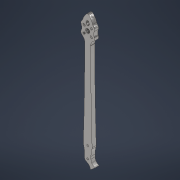
# Autodesk Inventor part: 10inchreararm
Saved by Autodesk Inventor 2021 (Build 250183000, 183)
## iProperties
Created: 2020-05-02
Part Number: 10inchreararm
Material: Generic
Document SubType Name: Modeling
Designer: Logan
Density: 1 g/cm^3
Appearance: Diamond Plate
Mass: 15.5755 g
Surface Area: 86.9393 cm^2
Volume: 15.5755 cm^3
Author: Logan
Autodesk Inventor part; units mm, degrees
ref_plane "YZ Plane" through (0, 0, 0) normal (1, 0, 0) x (0, 1, 0)
ref_plane "XZ Plane" through (0, 0, 0) normal (0, 1, 0) x (-1, 0, 0)
ref_plane "XY Plane" through (0, 0, 0) normal (0, 0, 1) x (1, 0, 0)
sketch "Sketch1" plane through (0, 0, 0) normal (0, 0, 1) x (1, 0, 0)
  line L0 (0, 0) -> (0, 20) construction
  line L1 (0, 20) -> (0, 190) construction
  line L2 (5, 20) -> (5, 190)
  line L3 (-5, 190) -> (-5, 20)
  arc A0 (-5, 20) -> (5, 20) centre (0, 20) ccw
  arc A1 (5, 190) -> (-5, 190) centre (0, 190) ccw
  line L4 (-6.7175, 196.7175) -> (6.7175, 183.2825) construction
  line L5 (-10.253, 193.182) -> (3.182, 179.747)
  line L6 (10.253, 186.818) -> (-3.182, 200.253)
  arc A2 (-3.182, 200.253) -> (-10.253, 193.182) centre (-6.7175, 196.7175) ccw
  arc A3 (3.182, 179.747) -> (10.253, 186.818) centre (6.7175, 183.2825) ccw
  line L7 (0, 190) -> (19, 190) construction
  line L8 (-6.7175, 183.2825) -> (6.7175, 196.7175) construction
  line L9 (-3.182, 179.747) -> (10.253, 193.182)
  line L10 (3.182, 200.253) -> (-10.253, 186.818)
  arc A4 (-10.253, 186.818) -> (-3.182, 179.747) centre (-6.7175, 183.2825) ccw
  arc A5 (10.253, 193.182) -> (3.182, 200.253) centre (6.7175, 196.7175) ccw
  line L11 (0, 190) -> (19, 190) construction
  line L12 (0, 190) -> (0, 212)
  arc A6 (6.7175, 196.7175) -> (0, 212) centre (-18.2146, 194.8761) ccw construction
  arc A7 (9.7094, 196.9385) -> (2.1857, 214.0549) centre (-18.2146, 194.8761) ccw
  arc A8 (3.7257, 196.4965) -> (-2.1857, 209.9451) centre (-18.2146, 194.8761) ccw
  arc A9 (3.7257, 196.4965) -> (9.7094, 196.9385) centre (6.7175, 196.7175) ccw
  arc A10 (2.1857, 214.0549) -> (-2.1857, 209.9451) centre (0, 212) ccw
  arc A11 (0, 212) -> (-6.7175, 196.7175) centre (18.2146, 194.8761) ccw construction
  arc A12 (-2.1857, 214.0549) -> (-9.7094, 196.9385) centre (18.2146, 194.8761) ccw
  arc A13 (2.1857, 209.9451) -> (-3.7257, 196.4965) centre (18.2146, 194.8761) ccw
  arc A14 (2.1857, 209.9451) -> (-2.1857, 214.0549) centre (0, 212) ccw
  arc A15 (-9.7094, 196.9385) -> (-3.7257, 196.4965) centre (-6.7175, 196.7175) ccw
  circle A16 centre (-6.7175, 196.7175) radius 1.5
  circle A17 centre (6.7175, 196.7175) radius 1.5
  circle A18 centre (6.7175, 183.2825) radius 1.5
  circle A19 centre (-6.7175, 183.2825) radius 1.5
  circle A20 centre (0, 190) radius 3.5
  circle A21 centre (0, 20) radius 1.5
  circle A22 centre (0, 0) radius 1.5
  circle A23 centre (0, 20) radius 7.5
  line L13 (0, 20) -> (0, 0) construction
  line L14 (-5.5, 20) -> (-5.5, 0)
  line L15 (5.5, 0) -> (5.5, 20)
  arc A24 (5.5, 20) -> (-5.5, 20) centre (0, 20) ccw
  arc A25 (-5.5, 0) -> (5.5, 0) centre (0, 0) ccw
  line L16 (0, 0) -> (17.3553, -20.6832)
  line L17 (0, 0) -> (27, 0) construction
  line L18 (8.6776, -10.3416) -> (12.5079, -7.1277)
  line L19 (8.6776, -10.3416) -> (4.8474, -13.5555)
  line L20 (8.6776, -10.3416) -> (13.6776, -10.3416) construction
  line L21 (0, 0) -> (3.8302, 3.2139)
  line L22 (0, 0) -> (5, 0) construction
  line L23 (0, 0) -> (-3.8302, -3.2139)
  line L24 (0, 0) -> (5, 0) construction
  arc A26 (4.8474, -13.5555) -> (-3.8302, -3.2139) centre (-7.0918, -14.7622) ccw
  arc A27 (3.8302, 3.2139) -> (12.5079, -7.1277) centre (15.7694, 4.4206) ccw
  line L25 (0, 190) -> (5.6569, 195.6569)
  circle A28 centre (5.6569, 195.6569) radius 1.5
  circle A29 centre (-5.6569, 195.6569) radius 1.5
  circle A30 centre (-5.6569, 184.3431) radius 1.5
  circle A31 centre (5.6569, 184.3431) radius 1.5
  point P0 (0, 10)
  point P1 (0, 105)
  point P2 (-7.0711, 190)
  point P3 (-5, 178.5867)
  point P4 (5, 178.5867)
  point P5 (7.0711, 190)
  point P6 (9.0793, 201.1245)
  point P7 (-2.1857, 214.0549)
  point P8 (-9.0793, 201.1245)
  point P9 (0, 197.0711)
  point P10 (-3.131, 200.2021)
  point P11 (0, 207.2142)
  point P12 (3.131, 200.2021)
  point P13 (0, 10)
  point P14 (-5, 25.5902)
  point P15 (-5.5, 14.901)
  point P16 (5.5, 14.901)
  point P17 (5, 25.5902)
  point P18 (5.3048, -1.4524)
  point P19 (0.5091, -5.4764)
  point P20 (-7.1057, 195.2686)
  point P21 (-5.2686, 197.1057)
  point P22 (-5.2686, 182.8943)
  point P23 (-7.1057, 184.7314)
  point P24 (7.1057, 184.7314)
  point P25 (5.2686, 182.8943)
  point P26 (5.2686, 197.1057)
  point P27 (7.1057, 195.2686)
  dimension "d15" = 3
  dimension "d16" = 3
  dimension "d17" = 3
  dimension "d18" = 3
  dimension "d0" = 20
  dimension "d2" = 170
  dimension "d3" = 10
  dimension "d4" = 9.5
  dimension "d5" = 45
  dimension "d6" = 10
  dimension "d7" = 9.5
  dimension "d8" = 45
  dimension "d9" = 10
  dimension "d10" = 22
  dimension "d11" = 25
  dimension "d12" = 6
  dimension "d13" = 25
  dimension "d14" = 6
  dimension "d19" = 7
  dimension "d20" = 3
  dimension "d21" = 3
  dimension "d27" = 15
  dimension "d28" = 11
  dimension "d29" = 27
  dimension "d30" = 50
  dimension "d31" = 5
  dimension "d33" = 5
  dimension "d35" = 5
  dimension "d36" = 40
  dimension "d37" = 5
  dimension "d38" = 140
  dimension "d39" = 12
  dimension "d40" = 12
  dimension "d41" = 90
  dimension "d42" = 90
  dimension "d43" = 8
  dimension "d44" = 3
  dimension "d45" = 3
  dimension "d46" = 3
  dimension "d47" = 3
  constraints: 62 end point, 40 point on circle, 28 centre point, 24 tangent, 9 coincident, 6 equal length, 6 horizontal, 6 midpoint, 4 parallel, 4 point on line, 3 vertical, 1 perpendicular, 12 other
  measures "d0" distance of L0.start L0.end
  measures "d2" distance of L0.end L1.end
  measures "d3" diameter of A1
  measures "d4" distance of L1.end L4.end
  measures "d5" angle of L4 L7
  measures "d6" diameter of A3
  measures "d7" distance of L1.end L8.end
  measures "d8" angle of L11 L8
  measures "d9" diameter of A5
  measures "d10" distance of L1.end L12.end
  measures "d11" radius of A6
  measures "d12" diameter of A9
  measures "d13" radius of A11
  measures "d14" diameter of A15
  measures "d19" diameter of A20
  measures "d20" diameter of A21
  measures "d21" diameter of A22
  measures "d27" diameter of A23
  measures "d28" diameter of A25
  measures "d29" distance of L13.end L16.end
  measures "d30" angle of L16 L17
  measures "d31" distance of L18.start L18.end
  measures "d33" distance of L18.start L19.end
  measures "d35" distance of L13.end L21.end
  measures "d36" angle of L22 L21
  measures "d37" distance of L13.end L23.end
  measures "d38" angle of L23 L24
  measures "d39" radius of A26
  measures "d40" radius of A27
  measures "d41" angle of L16 L18
  measures "d42" angle of L16 L19
  measures "d43" distance of L25.start L25.end
  measures "d44" diameter of A28
  measures "d45" diameter of A29
  measures "d46" diameter of A30
  measures "d47" diameter of A31
extrude "Extrusion1" add sketch "Sketch1" along normal blind 7 contours A0 L3 A24 L2 | L2 A24 L15 A23 L14 L3 A0 | A24 L3 A23 L2 | L2 A23 L15 A24 | A23 L3 A4 L9 L5 A3 L2 | A24 L14 A23 L3 | A3 L5 L9 L2 A31 | L2 A31 A18 L9 L6 A3 | L15 A25 A27 L21 A22 L23 A26 L14 A23 | A4 L10 L5 L3 A30 A19 | L3 A30 L5 L9 A4 | L5 L3 A1 L12 A20 L25 L2 L9 | L9 L2 A1 L6 | L6 L25 A9 A7 A5 L9 | A27 L18 L16 A25 | A25 L16 A22 L21 A27 | L5 L10 A1 L3 | L25 A20 L12 A1 | A1 L12 L6 | L6 L10 A8 A9 L25 | L5 A2 A12 A15 A13 L6 L10 | A26 L23 A22 L16 A25 | A25 L16 L19 A26 | A1 L10 L12 | A9 A8 L10 A5 A7 | A5 L10 A8 A13 A14 A7 | A13 A15 A12 A2 L6 | L6 A2 A12 A10 A8 A13 | A8 A10 A14 A13
fillet "Fillet1" radius 4500 2 edges at (5, 25.5902, 3.5) (-5, 25.5902, 3.5)
fillet "Fillet2" radius 10 8 edges at (-9.0793, 201.1245, 3.5) (-7.0711, 190, 3.5) (-5, 178.5867, 3.5) (5, 178.5867, 3.5) (7.0711, 190, 3.5) (9.0793, 201.1245, 3.5) (5.3048, -1.4524, 3.5) (0.5091, -5.4764, 3.5)
fillet "Fillet3" radius 1.6 4 edges at (0, 207.2142, 3.5) (-3.131, 200.2021, 3.5) (0, 197.0711, 3.5) (3.131, 200.2021, 3.5)
fillet "Fillet4" radius 40 2 edges at (5.5, 14.901, 3.5) (-5.5, 14.901, 3.5)
body "Solid1"
